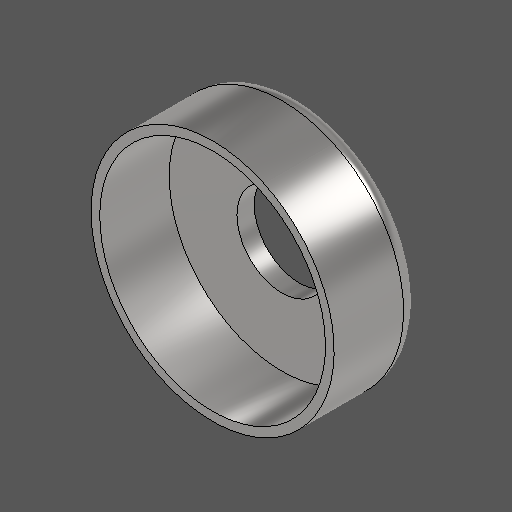
# Autodesk Inventor part: Electrode Skirt Short
Saved by Autodesk Inventor 2025 (Build 290162000, 162)
## iProperties
Created: 2024-05-18
Part Number: Electrode Skirt Short
Material: Stainless Steel
Document SubType Name: Modeling
Designer: KAA
Density: 8 g/cm^3
Appearance: Semi-Polished
Mass: 1.29421 g
Surface Area: 6.77265 cm^2
Volume: 0.161776 cm^3
Author: KAA
Title: Electrod Skirt Short
Autodesk Inventor part; units mm, degrees
ref_plane "YZ Plane" through (0, 0, 0) normal (1, 0, 0) x (0, 1, 0)
ref_plane "XZ Plane" through (0, 0, 0) normal (0, 1, 0) x (-1, 0, 0)
ref_plane "XY Plane" through (0, 0, 0) normal (0, 0, 1) x (1, 0, 0)
sketch "Sketch3" plane through (0, 0, 0) normal (1, 0, 0) x (0, 1, 0)
  line L0 (0, 0) -> (0, 24.2821)
  line L1 (7, 0) -> (7, 5)
  line L2 (7, 5) -> (6.5, 5)
  line L3 (6.5, 5) -> (6.5, 1)
  line L4 (6.5, 1) -> (2.6, 1)
  line L5 (2.6, 1) -> (2.6, 0)
  line L6 (7, 0) -> (2.6, 0)
  dimension "d7" = 5.2
  dimension "d10" = 1
  dimension "d12" = 5
  dimension "d13" = 14
  dimension "d14" = 13
  constraints: 14 end point, 3 perpendicular, 1 horizontal, 1 horizontal alignment, 1 vertical
  measures "d7" diameter of L5 L0
  measures "d10" distance of L4.end L5.end
  measures "d12" distance of L1.start L1.end
  measures "d13" diameter of L1 L0
  measures "d14" diameter of L3 L0
revolve "Revolution1" add sketch "Sketch3" angle 360 about axis through (0, 0, 0) along (0, 0, 1)
fillet "Fillet1" radius 1 1 edges at (0, -7, 0)
equation "\"d10\" = wall_thickness"
equation "\"wall_thickness\" = 1"
body "Solid2"
